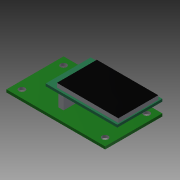
# Autodesk Inventor part: LCD-RTC
Saved by Autodesk Inventor 2015 (Build 190159000, 159)
## iProperties
Created: 2016-04-26
Part Number: LCD-RTC
Material: 一般
Document SubType Name: Modeling
Designer: yamashita1
Density: 1 g/cm^3
Appearance: 既定
Author: yamashita1
Autodesk Inventor part; units mm, degrees
ref_plane "YZ Plane" through (0, 0, 0) normal (1, 0, 0) x (0, 1, 0)
ref_plane "XZ Plane" through (0, 0, 0) normal (0, 1, 0) x (-1, 0, 0)
ref_plane "XY Plane" through (0, 0, 0) normal (0, 0, 1) x (1, 0, 0)
sketch "スケッチ1" plane through (0, 0, 0) normal (0, 0, 1) x (1, 0, 0)
  line L0 (-24.13, -13.97) -> (24.13, -13.97)
  line L1 (24.13, -13.97) -> (24.13, 13.97)
  line L2 (24.13, 13.97) -> (-24.13, 13.97)
  line L3 (-24.13, 13.97) -> (-24.13, -13.97)
  point P0 (0, 0)
  point P1 (0, -13.97)
  point P2 (24.13, 0)
  dimension "d0" = 48.26
  dimension "d1" = 27.94
  constraints: 8 end point, 2 midpoint, 2 parallel, 1 horizontal, 1 horizontal alignment, 1 perpendicular, 1 vertical alignment
  measures "d0" distance of L2.end L1.end
  measures "d1" distance of L1.end L0.end
extrude "押し出し1" add sketch "スケッチ1" along normal blind 1.3
sketch "スケッチ2" plane through (0, 0, 1.3) normal (0, 0, 1) x (1, 0, 0)
  line L0 (-24.13, 13.97) -> (-24.13, -13.97) projected
  line L1 (24.13, 13.97) -> (-24.13, 13.97) projected
  line L2 (-24.13, -13.97) -> (24.13, -13.97) projected
  line L3 (24.13, -13.97) -> (24.13, 13.97) projected
  circle A0 centre (-20.32, 10.16) radius 1.5
  circle A1 centre (-20.32, -10.16) radius 1.5
  circle A2 centre (20.32, -10.16) radius 1.5
  circle A3 centre (20.32, 10.16) radius 1.5
  point P0 (0, 0)
  dimension "d4" = 3.81
  dimension "d5" = 3.81
  dimension "d6" = 3.81
  dimension "d7" = 3.81
  dimension "d8" = 3
  constraints: 4 centre point, 4 coincident, 3 equal radius, 2 horizontal alignment, 2 vertical alignment
  measures "d4" distance from line of L0 point (-20.32, 10.16)
  measures "d5" distance from line of L1 point (-20.32, 10.16)
  measures "d6" distance from line of L2 point (-20.32, -10.16)
  measures "d7" distance from line of point (20.32, 10.16) L3
  measures "d8" diameter of A0
extrude "押し出し2" cut sketch "スケッチ2" against normal blind 1.3 contours A0 | A1 | A2 | A3
sketch "スケッチ3" plane through (0, 0, 1.3) normal (0, 0, 1) x (1, 0, 0)
  circle A0 centre (-20.32, -10.16) radius 1.5 projected
  line L0 (-1.27, -8.89) -> (-3.81, -8.89)
  line L1 (-3.81, -8.89) -> (-3.81, 3.81)
  line L2 (-3.81, 3.81) -> (-1.27, 3.81)
  line L3 (-1.27, 3.81) -> (-1.27, -8.89)
  point P0 (0, 0)
  point P1 (-2.54, -7.62)
  point P2 (-2.54, -8.89)
  dimension "d11" = 17.78
  dimension "d12" = 2.54
  dimension "d13" = 2.54
  dimension "d14" = 12.7
  dimension "d15" = 1.27
  constraints: 8 end point, 2 parallel, 1 horizontal, 1 midpoint, 1 perpendicular, 1 vertical alignment
  measures "d11" horizontal distance of A0.centre point (-2.54, -7.62)
  measures "d12" vertical distance of A0.centre point (-2.54, -7.62)
  measures "d13" distance of L1.end L2.end
  measures "d14" distance of L0.end L1.end
  measures "d15" distance of point (-2.54, -7.62) point (-2.54, -8.89)
extrude "押し出し3" add sketch "スケッチ3" along normal blind 8.5 contours L0 L1 L2 L3
sketch "スケッチ4" plane through (0, 0, 9.8) normal (0, 0, 1) x (1, 0, 0)
  line L0 (-3.81, 3.81) -> (-1.27, 3.81)
  line L1 (-1.27, 3.81) -> (-1.27, -8.89)
  line L2 (-1.27, -8.89) -> (-3.81, -8.89)
  line L3 (-3.81, -8.89) -> (-3.81, 3.81)
  point P0 (0, 0)
  constraints: 8 end point, 2 parallel, 1 horizontal, 1 perpendicular
extrude "押し出し4" add sketch "スケッチ4" along normal blind 2
sketch "スケッチ5" plane through (0, 0, 11.8) normal (0, 0, 1) x (1, 0, 0)
  line L0 (-5.35, 8.46) -> (29.65, 8.46)
  line L1 (29.65, 8.46) -> (29.65, -13.54)
  line L2 (29.65, -13.54) -> (-5.35, -13.54)
  line L3 (-5.35, -13.54) -> (-5.35, 8.46)
  line L4 (-3.81, 3.81) -> (-3.81, -8.89) projected
  point P0 (0, 0)
  point P1 (-5.35, -2.54)
  point P2 (-3.81, -2.54)
  dimension "d20" = 35
  dimension "d21" = 22
  dimension "d22" = 1.54
  constraints: 8 end point, 2 midpoint, 2 parallel, 1 horizontal, 1 horizontal alignment, 1 perpendicular
  measures "d20" distance of L1.end L2.end
  measures "d21" distance of L0.end L1.end
  measures "d22" horizontal distance of L4.end L2.end
extrude "押し出し5" add sketch "スケッチ5" along normal blind 1.2
sketch "スケッチ6" plane through (0, 0, 13) normal (0, 0, 1) x (1, 0, 0)
  line L0 (29.15, 6.96) -> (-0.85, 6.96)
  line L1 (-0.85, 6.96) -> (-0.85, -12.54)
  line L2 (-0.85, -12.54) -> (29.15, -12.54)
  line L3 (29.15, -12.54) -> (29.15, 6.96)
  line L4 (29.65, -13.54) -> (29.65, 8.46) projected
  point P0 (0, 0)
  dimension "d25" = 30
  dimension "d26" = 19.5
  dimension "d27" = 0.5
  dimension "d28" = 1
  constraints: 8 end point, 2 parallel, 1 horizontal, 1 perpendicular
  measures "d25" distance of L2.end L1.end
  measures "d26" distance of L1.end L0.end
  measures "d27" distance from line of L4 L2.end
  measures "d28" vertical distance of L4.start L2.end
extrude "押し出し6" add sketch "スケッチ6" along normal blind 2
